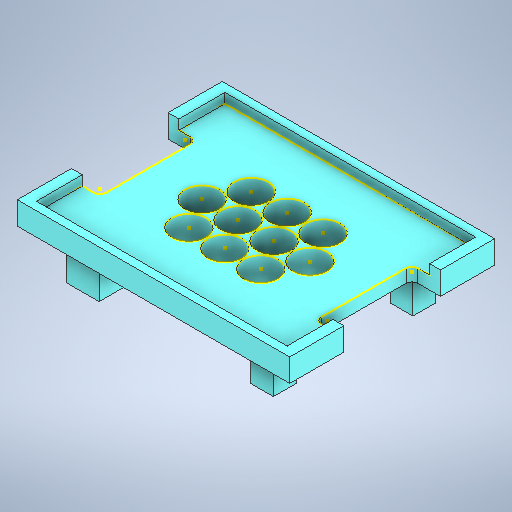
# Autodesk Inventor part: PILLARSCELLCASE18650
Saved by Autodesk Inventor 2025.2 (Build 292293000, 293)
## iProperties
Created: 2024-11-21
Part Number: PILLARSCELLCASE18650
Material: Generic
Document SubType Name: Modeling
Designer: cbast
Density: 1 g/cm^3
Appearance: Default
Mass: 190.937 g
Surface Area: 666.623 cm^2
Volume: 190.937 cm^3
Author: cbast
## iProperties of the stored document BatteryCasev1_3DPrint.ipt
Created: 2025-01-30
Part Number: BatteryCasev1_3DPrint
Material: Generic
Document SubType Name: Modeling
Designer: cbast
Density: 1 g/cm^3
Appearance: Default
Author: cbast
Autodesk Inventor part; units mm, degrees
ref_plane "YZ Plane" through (0, 0, 0) normal (1, 0, 0) x (0, 1, 0)
ref_plane "XZ Plane" through (0, 0, 0) normal (0, 1, 0) x (-1, 0, 0)
ref_plane "XY Plane" through (0, 0, 0) normal (0, 0, 1) x (1, 0, 0)
sketch "Sketch1" plane through (0, 0, 0) normal (0, 1, 0) x (-1, 0, 0)
  circle A0 centre (0, 0) radius 10.5
  circle A1 centre (22, 0) radius 10.5
  circle A2 centre (-22, 0) radius 10.5
  circle A3 centre (-11, 19.0526) radius 10.5
  circle A4 centre (11, 19.0526) radius 10.5
  circle A5 centre (33, 19.0526) radius 10.5
  circle A6 centre (11, -19.0526) radius 10.5
  circle A7 centre (33, -19.0526) radius 10.5
  circle A8 centre (-11, -19.0526) radius 10.5
  circle A9 centre (44, 0) radius 10.5
  line L0 (0, 0) -> (-32.9562, 0) construction
  line L1 (-32.9562, 0) -> (61.076, 0) construction
  circle A10 centre (0, 0) radius 11.5 construction
  circle A11 centre (-22, 0) radius 11.5 construction
  circle A12 centre (-11, -19.0526) radius 11.5 construction
  circle A13 centre (11, -19.0526) radius 11.5 construction
  circle A14 centre (33, -19.0526) radius 11.5 construction
  circle A15 centre (44, 0) radius 11.5 construction
  circle A16 centre (22, 0) radius 11.5 construction
  circle A17 centre (33, 19.0526) radius 11.5 construction
  circle A18 centre (11, 19.0526) radius 11.5 construction
  circle A19 centre (-11, 19.0526) radius 11.5 construction
  circle A20 centre (44, 0) radius 12.5 construction
  circle A21 centre (33, -19.0526) radius 12.5 construction
  circle A22 centre (11, -19.0526) radius 12.5 construction
  circle A23 centre (-11, -19.0526) radius 12.5 construction
  circle A24 centre (-22, 0) radius 12.5 construction
  circle A25 centre (-11, 19.0526) radius 12.5 construction
  circle A26 centre (11, 19.0526) radius 12.5 construction
  circle A27 centre (33, 19.0526) radius 12.5 construction
  circle A28 centre (0, 0) radius 12.5 construction
  circle A29 centre (22, 0) radius 12.5 construction
  arc A30 (43.6417, -12.4949) -> (43.6417, 12.4949) centre (43.6417, 0) ccw
  arc A31 (43.6417, 12.4949) -> (22, 24.9897) centre (33, 19.0526) ccw
  arc A32 (22, 24.9897) -> (0, 24.9897) centre (11, 19.0526) ccw
  arc A33 (0, 24.9897) -> (-21.6417, 12.4949) centre (-11, 19.0526) ccw
  arc A34 (-21.6417, 12.4949) -> (-21.6417, -12.4949) centre (-22, 0) ccw
  arc A35 (-21.6417, -12.4949) -> (0, -24.9897) centre (-11, -19.0526) ccw
  arc A36 (0, -24.9897) -> (22, -24.9897) centre (11, -19.0526) ccw
  arc A37 (22, -24.9897) -> (43.6417, -12.4949) centre (33, -19.0526) ccw
  point P0 (28.893, 7.4235)
  dimension "d0" = 21
  dimension "d2" = 21
  dimension "d4" = 21
  dimension "d6" = 21
  dimension "d8" = 21
  dimension "d10" = 21
  dimension "d11" = 21
  dimension "d13" = 21
  dimension "d14" = 21
  dimension "d53" = 21
  dimension "d91" = 1
  dimension "d144" = 23
  dimension "d145" = 23
  dimension "d146" = 23
  dimension "d147" = 23
  dimension "d148" = 23
  dimension "d149" = 23
  dimension "d150" = 23
  dimension "d151" = 23
  dimension "d152" = 23
  dimension "d153" = 23
  dimension "d154" = 25
  dimension "d155" = 25
  dimension "d156" = 25
  dimension "d157" = 25
  dimension "d158" = 25
  dimension "d159" = 25
  dimension "d160" = 25
  dimension "d161" = 25
  dimension "d162" = 25
  dimension "d163" = 25
  constraints: 38 centre point, 32 point on circle, 22 coincident, 16 tangent, 9 concentric, 4 end point, 2 point on line, 1 horizontal
  measures "d0" diameter of A0
  measures "d2" diameter of A1
  measures "d4" diameter of A2
  measures "d6" diameter of A3
  measures "d8" diameter of A4
  measures "d10" diameter of A5
  measures "d11" diameter of A6
  measures "d13" diameter of A7
  measures "d14" diameter of A8
  measures "d53" diameter of A9
  measures "d144" diameter of A10
  measures "d145" diameter of A11
  measures "d146" diameter of A12
  measures "d147" diameter of A13
  measures "d148" diameter of A14
  measures "d149" diameter of A15
  measures "d150" diameter of A16
  measures "d151" diameter of A17
  measures "d152" diameter of A18
  measures "d153" diameter of A19
  measures "d154" diameter of A20
  measures "d155" diameter of A21
  measures "d156" diameter of A22
  measures "d157" diameter of A23
  measures "d158" diameter of A24
  measures "d159" diameter of A25
  measures "d160" diameter of A26
  measures "d161" diameter of A27
  measures "d162" diameter of A28
  measures "d163" diameter of A29
extrude "Extrusion1" add sketch "Sketch1" along normal blind 15
sketch "Sketch4" plane through (0, 15, 0) normal (0, 1, 0) x (1, 0, 0)
  circle A0 centre (-33, 19.0526) radius 10.5 projected
  circle A1 centre (-44, 0) radius 10.5 projected
  circle A2 centre (-44, 0) radius 10.5 projected
  circle A3 centre (11, 19.0526) radius 10.5 projected
  circle A4 centre (-33, 19.0526) radius 10.5 projected
  circle A5 centre (-11, 19.0526) radius 10.5 projected
  circle A6 centre (-33, -19.0526) radius 10.5 projected
  circle A7 centre (-11, -19.0526) radius 10.5 projected
  circle A8 centre (11, -19.0526) radius 10.5 projected
  circle A9 centre (22, 0) radius 10.5 projected
  circle A10 centre (-22, 0) radius 10.5 projected
  circle A11 centre (0, 0) radius 10.5 projected
  line L0 (0, 0) -> (-11, 0) construction
  line L1 (-87.7, 57.7) -> (65.7, 57.7)
  line L2 (65.7, 57.7) -> (65.7, -57.7)
  line L3 (65.7, -57.7) -> (-87.7, -57.7)
  line L4 (-87.7, -57.7) -> (-87.7, 57.7)
  line L5 (-87.7, 57.7) -> (65.7, -57.7) construction
  line L6 (65.7, 57.7) -> (-87.7, -57.7) construction
  arc A12 (0, 24.9897) -> (-22, 24.9897) centre (-11, 19.0526) ccw projected
  arc A13 (21.6417, 12.4949) -> (0, 24.9897) centre (11, 19.0526) ccw projected
  arc A14 (21.6417, -12.4949) -> (21.6417, 12.4949) centre (22, 0) ccw projected
  arc A15 (0, -24.9897) -> (21.6417, -12.4949) centre (11, -19.0526) ccw projected
  arc A16 (-22, -24.9897) -> (0, -24.9897) centre (-11, -19.0526) ccw projected
  arc A17 (-43.6417, -12.4949) -> (-22, -24.9897) centre (-33, -19.0526) ccw projected
  circle A18 centre (-33, 19.0526) radius 12.5 construction
  arc A19 (-43.6417, 12.4949) -> (-43.6417, -12.4949) centre (-43.6417, 0) ccw projected
  arc A20 (-22, 24.9897) -> (-43.6417, 12.4949) centre (-33, 19.0526) ccw projected
  arc A21 (0, 24.9897) -> (-22, 24.9897) centre (-11, 19.0526) ccw
  arc A22 (21.6417, 12.4949) -> (0, 24.9897) centre (11, 19.0526) ccw
  arc A23 (21.6417, -12.4949) -> (21.6417, 12.4949) centre (22, 0) ccw
  arc A24 (0, -24.9897) -> (21.6417, -12.4949) centre (11, -19.0526) ccw
  arc A25 (-22, -24.9897) -> (0, -24.9897) centre (-11, -19.0526) ccw
  arc A26 (-43.6417, -12.4949) -> (-22, -24.9897) centre (-33, -19.0526) ccw
  arc A27 (-43.6417, 12.4949) -> (-43.6417, -12.4949) centre (-43.6417, 0) ccw
  arc A28 (-22, 24.9897) -> (-43.6417, 12.4949) centre (-33, 19.0526) ccw
  line L7 (-11.5, 0) -> (-10.5, 0) construction
  point P0 (-17.0502, -21.4927)
  point P1 (-17.0502, -11.5134)
  point P2 (-17.0502, -8.8009)
  point P3 (-17.0502, 8.8009)
  point P4 (-17.0502, 11.5134)
  point P5 (-17.0502, 21.4927)
  point P6 (-2.0059, 21.4927)
  point P7 (-2.0059, -11.5134)
  point P8 (-2.0059, -8.8009)
  point P9 (-2.0059, 8.8009)
  point P10 (-2.0059, 11.5134)
  point P11 (-2.0059, -21.4927)
  dimension "d104" = 153.4
  dimension "d164" = 115.4
  constraints: 16 end point, 16 point on circle, 8 centre point, 8 concentric, 3 midpoint, 2 horizontal, 2 parallel, 1 perpendicular, 1 point on line, 4 other
  measures "d104" distance of L2.end L3.end
  measures "d164" distance of L1.end L2.end
extrude "Extrusion7" add sketch "Sketch4" against normal blind 8 contours L1 L2 L3 L4
sketch "Sketch5" plane through (0, 15, 0) normal (0, 1, 0) x (1, 0, 0)
  line L0 (-87.7, -57.7) -> (65.7, -57.7) projected
  line L1 (65.7, -57.7) -> (65.7, 57.7) projected
  line L2 (65.7, 57.7) -> (-87.7, 57.7) projected
  line L3 (-87.7, 57.7) -> (-87.7, -57.7) projected
  circle A0 centre (-44, 0) radius 10.5 projected
  circle A1 centre (11, 19.0526) radius 10.5 projected
  circle A2 centre (-33, 19.0526) radius 10.5 projected
  circle A3 centre (-11, 19.0526) radius 10.5 projected
  circle A4 centre (-33, -19.0526) radius 10.5 projected
  circle A5 centre (-11, -19.0526) radius 10.5 projected
  circle A6 centre (11, -19.0526) radius 10.5 projected
  circle A7 centre (22, 0) radius 10.5 projected
  circle A8 centre (-22, 0) radius 10.5 projected
  circle A9 centre (0, 0) radius 10.5 projected
  line L4 (-87.7, 57.7) -> (65.7, 57.7)
  line L5 (65.7, 57.7) -> (65.7, -57.7)
  line L6 (65.7, -57.7) -> (-87.7, -57.7)
  line L7 (-87.7, -57.7) -> (-87.7, 57.7)
  line L8 (-94.3464, -62.7) -> (72.3464, -62.7)
  line L9 (72.3464, -62.7) -> (72.3464, 62.7)
  line L10 (72.3464, 62.7) -> (-94.3464, 62.7)
  line L11 (-94.3464, 62.7) -> (-94.3464, -62.7)
  line L12 (-94.3464, -62.7) -> (72.3464, 62.7) construction
  line L13 (72.3464, -62.7) -> (-94.3464, 62.7) construction
  point P0 (66.922, -57.45)
  point P1 (-11, 0)
  dimension "d169" = 5
  dimension "d170" = 6.6464
  dimension "d171" = 166.6929
  dimension "d172" = 125.4
  dimension "d221" = 6.6464
  constraints: 20 end point, 4 parallel, 4 point on line, 2 horizontal, 2 midpoint, 2 perpendicular
  measures "d169" distance between parallel lines of L10 L4
  measures "d170" distance between parallel lines of L9 L5
  measures "d171" distance of L9.end L10.end
  measures "d172" distance of L10.end L8.start
  measures "d221" distance between parallel lines of L3 L11
extrude "Extrusion8" add sketch "Sketch5" along normal blind 6 and the other way blind 8 contours L11 L10 L9 L8
sketch "Sketch6" plane through (0, 15, 0) normal (0, 1, 0) x (1, 0, 0)
  line L0 (58.472, 57.1514) -> (58.472, 25.95) construction
  line L1 (58.472, 25.95) -> (65.7, 25.95) construction
  line L2 (-80.472, -57.7) -> (-80.472, -25.95) construction
  line L3 (-80.472, -25.95) -> (-87.7, -25.95) construction
  circle A0 centre (58.472, 25.95) radius 3.615
  circle A1 centre (58.472, -25.95) radius 3.615
  circle A2 centre (-80.472, -25.95) radius 3.615
  circle A3 centre (-80.472, 25.95) radius 3.615
  line L4 (72.3464, -62.7) -> (72.3464, 62.7) projected
  line L5 (72.3464, 62.7) -> (-94.3464, 62.7) projected
  line L6 (-94.3464, 62.7) -> (-94.3464, -62.7) projected
  line L7 (-94.3464, -62.7) -> (72.3464, -62.7) projected
  line L8 (-87.7, -57.7) -> (-87.7, 57.7) projected
  line L9 (-87.7, 57.7) -> (65.7, 57.7) projected
  line L10 (65.7, 57.7) -> (65.7, -57.7) projected
  line L11 (65.7, -57.7) -> (-87.7, -57.7) projected
  line L12 (-87.7, -57.7) -> (65.7, -57.7) projected
  line L13 (65.7, -57.7) -> (65.7, 57.7) projected
  line L14 (65.7, 57.7) -> (-87.7, 57.7) projected
  line L15 (-87.7, 57.7) -> (-87.7, -57.7) projected
  circle A4 centre (-44, 0) radius 10.5 projected
  circle A5 centre (11, 19.0526) radius 10.5 projected
  circle A6 centre (-33, 19.0526) radius 10.5 projected
  circle A7 centre (-11, 19.0526) radius 10.5 projected
  circle A8 centre (-33, -19.0526) radius 10.5 projected
  circle A9 centre (-11, -19.0526) radius 10.5 projected
  circle A10 centre (11, -19.0526) radius 10.5 projected
  circle A11 centre (22, 0) radius 10.5 projected
  circle A12 centre (-22, 0) radius 10.5 projected
  circle A13 centre (0, 0) radius 10.5 projected
  line L16 (-87.7, 57.7) -> (65.7, 57.7)
  line L17 (65.7, 57.7) -> (65.7, -57.7)
  line L18 (65.7, -57.7) -> (-87.7, -57.7)
  line L19 (-87.7, -57.7) -> (-87.7, 57.7)
  dimension "d123" = 7.23
  dimension "d124" = 7.23
  dimension "d125" = 7.23
  dimension "d140" = 7.23
  dimension "d179" = 31.75
  dimension "d180" = 7.228
  dimension "d181" = 7.228
  dimension "d182" = 31.75
  dimension "d183" = 31.75
  dimension "d184" = 7.228
  dimension "d185" = 7.228
  dimension "d186" = 31.75
  constraints: 16 end point, 4 centre point, 2 coincident, 2 parallel, 1 horizontal, 1 perpendicular
  measures "d123" diameter of A0
  measures "d124" diameter of A1
  measures "d125" diameter of A2
  measures "d140" diameter of A3
  measures "d179" distance from line of A3.centre L16
  measures "d180" distance from line of A3.centre L15
  measures "d181" distance from line of A2.centre L8
  measures "d182" distance from line of L2.end L18
  measures "d183" distance from line of L12 A1.centre
  measures "d184" distance from line of L17 A1.centre
  measures "d185" distance from line of L17 L0.end
  measures "d186" distance from line of L16 L0.end
extrude "Extrusion6" cut sketch "Sketch6" against normal through all contours A0 | A1 | A2 | A3
sketch "Sketch7" plane through (-94.3464, 7, 62.7) normal (-1, 0, 0) x (0, 0, 1)
  line L0 (-120.4, 8) -> (-5, 8) projected
  line L1 (0, 0) -> (-125.4, 0) projected
  line L2 (-125.4, 14) -> (0, 14) projected
  line L3 (-92.265, 8) -> (-85.035, 8) projected
  line L4 (-40.365, 8) -> (-33.135, 8) projected
  line L5 (-92.265, 8) -> (-33.135, 8)
  line L6 (-33.135, 8) -> (-33.135, 14)
  line L7 (-33.135, 14) -> (-92.265, 14)
  line L8 (-92.265, 14) -> (-92.265, 8)
  point P0 (-62.7, -7)
  constraints: 8 end point, 2 parallel, 1 horizontal, 1 perpendicular, 1 point on line
extrude "Extrusion9" cut sketch "Sketch7" against normal through all
sketch "Sketch10" plane through (0, 7, 0) normal (0, -1, 0) x (1, 0, 0)
  circle A0 centre (-80.472, 25.95) radius 3.615 projected
  circle A1 centre (58.472, 25.95) radius 3.615 projected
  circle A2 centre (-80.472, -25.95) radius 3.615 projected
  circle A3 centre (58.472, -25.95) radius 3.615 projected
  line L0 (72.3464, -62.7) -> (72.3464, 62.7) projected
  line L1 (72.3464, 62.7) -> (-94.3464, 62.7) projected
  line L2 (-94.3464, 62.7) -> (-94.3464, -62.7) projected
  line L3 (-94.3464, -62.7) -> (72.3464, -62.7) projected
  arc A4 (-43.6417, -12.4949) -> (-22, -24.9897) centre (-33, -19.0526) ccw projected
  arc A5 (-43.6417, 12.4949) -> (-43.6417, -12.4949) centre (-43.6417, 0) ccw projected
  arc A6 (-22, 24.9897) -> (-43.6417, 12.4949) centre (-33, 19.0526) ccw projected
  arc A7 (0, 24.9897) -> (-22, 24.9897) centre (-11, 19.0526) ccw projected
  arc A8 (21.6417, 12.4949) -> (0, 24.9897) centre (11, 19.0526) ccw projected
  arc A9 (21.6417, -12.4949) -> (21.6417, 12.4949) centre (22, 0) ccw projected
  arc A10 (0, -24.9897) -> (21.6417, -12.4949) centre (11, -19.0526) ccw projected
  arc A11 (-22, -24.9897) -> (0, -24.9897) centre (-11, -19.0526) ccw projected
  line L4 (-94.3464, 62.7) -> (-64.3464, 62.7) construction
  line L5 (-94.3464, 62.7) -> (-94.3464, 42.7) construction
  line L6 (-94.3464, 42.7) -> (-64.3464, 42.7) construction
  line L7 (-74.3464, 52.7) -> (-54.3464, 52.7)
  line L8 (-54.3464, 52.7) -> (-54.3464, 32.7)
  line L9 (-54.3464, 32.7) -> (-74.3464, 32.7)
  line L10 (-74.3464, 32.7) -> (-74.3464, 52.7)
  line L11 (-74.3464, 52.7) -> (-54.3464, 32.7) construction
  line L12 (-54.3464, 52.7) -> (-74.3464, 32.7) construction
  line L13 (-71.8464, 50.2) -> (-56.8464, 50.2)
  line L14 (-56.8464, 50.2) -> (-56.8464, 35.2)
  line L15 (-56.8464, 35.2) -> (-71.8464, 35.2)
  line L16 (-71.8464, 35.2) -> (-71.8464, 50.2)
  line L17 (-71.8464, 50.2) -> (-56.8464, 35.2) construction
  line L18 (-56.8464, 50.2) -> (-71.8464, 35.2) construction
  line L19 (-94.3464, 0) -> (72.3464, 0) construction
  line L20 (-74.3464, -52.7) -> (-54.3464, -52.7)
  line L21 (-54.3464, -52.7) -> (-54.3464, -32.7)
  line L22 (-54.3464, -32.7) -> (-74.3464, -32.7)
  line L23 (-74.3464, -32.7) -> (-74.3464, -52.7)
  line L24 (-74.3464, -52.7) -> (-54.3464, -32.7) construction
  line L25 (-54.3464, -52.7) -> (-74.3464, -32.7) construction
  line L26 (-71.8464, -50.2) -> (-56.8464, -50.2)
  line L27 (-56.8464, -50.2) -> (-56.8464, -35.2)
  line L28 (-56.8464, -35.2) -> (-71.8464, -35.2)
  line L29 (-71.8464, -35.2) -> (-71.8464, -50.2)
  line L30 (-71.8464, -50.2) -> (-56.8464, -35.2) construction
  line L31 (-56.8464, -50.2) -> (-71.8464, -35.2) construction
  line L32 (72.3464, 62.7) -> (42.3464, 62.7) construction
  line L33 (42.3464, 62.7) -> (42.3464, 42.7) construction
  line L34 (35.3464, 49.7) -> (49.3464, 49.7)
  line L35 (49.3464, 49.7) -> (49.3464, 35.7)
  line L36 (49.3464, 35.7) -> (35.3464, 35.7)
  line L37 (35.3464, 35.7) -> (35.3464, 49.7)
  line L38 (35.3464, 49.7) -> (49.3464, 35.7) construction
  line L39 (49.3464, 49.7) -> (35.3464, 35.7) construction
  line L40 (35.3464, -49.7) -> (49.3464, -49.7)
  line L41 (49.3464, -49.7) -> (49.3464, -35.7)
  line L42 (49.3464, -35.7) -> (35.3464, -35.7)
  line L43 (35.3464, -35.7) -> (35.3464, -49.7)
  line L44 (35.3464, -49.7) -> (49.3464, -35.7) construction
  line L45 (49.3464, -49.7) -> (35.3464, -35.7) construction
  line L46 (42.3464, -42.7) -> (42.3464, -62.7) construction
  line L47 (42.3464, -42.7) -> (72.3464, -42.7) construction
  line L48 (-64.3464, -42.7) -> (-64.3464, -62.7) construction
  line L49 (-64.3464, -42.7) -> (-94.3464, -42.7) construction
  point P0 (0, 0)
  dimension "d209" = 30
  dimension "d210" = 20
  dimension "d211" = 20
  dimension "d212" = 20
  dimension "d213" = 15
  dimension "d214" = 15
  dimension "d215" = 30
  dimension "d216" = 20
  dimension "d217" = 14
  dimension "d218" = 14
  dimension "d224" = 30
  dimension "d225" = 30
  dimension "d226" = 20
  dimension "d227" = 20
  constraints: 92 end point, 14 symmetric about line, 8 midpoint, 8 point on line, 7 parallel, 6 perpendicular, 4 horizontal
  measures "d209" distance of L1.end L4.end
  measures "d210" distance of L1.end L5.end
  measures "d211" distance of L8.end L9.end
  measures "d212" distance of L7.end L8.end
  measures "d213" distance of L14.end L15.end
  measures "d214" distance of L13.end L14.end
  measures "d215" distance of L0.end L32.end
  measures "d216" distance of L32.end L33.end
  measures "d217" distance of L35.end L36.end
  measures "d218" distance of L34.end L35.end
  measures "d224" distance of L48.start L49.end
  measures "d225" distance of L46.start L47.end
  measures "d226" distance of L46.start L46.end
  measures "d227" distance of L48.start L48.end
extrude "Extrusion11" add sketch "Sketch10" along normal blind 25 contours L7 L8 L9 L10 | L23 L22 L21 L20 | L34 L35 L36 L37 | L43 L42 L41 L40
sketch "Sketch11" plane through (0, 7, 0) normal (0, -1, 0) x (1, 0, 0)
  line L0 (-71.8464, 50.2) -> (-71.8464, 35.2) projected
  line L1 (-71.8464, 35.2) -> (-56.8464, 35.2) projected
  line L2 (-56.8464, 35.2) -> (-56.8464, 50.2) projected
  line L3 (-56.8464, 50.2) -> (-71.8464, 50.2) projected
  line L4 (-71.8464, 50.2) -> (-56.8464, 50.2)
  line L5 (-56.8464, 50.2) -> (-56.8464, 35.2)
  line L6 (-56.8464, 35.2) -> (-71.8464, 35.2)
  line L7 (-71.8464, 35.2) -> (-71.8464, 50.2)
  line L8 (-56.8464, -35.2) -> (-71.8464, -35.2) projected
  line L9 (-71.8464, -35.2) -> (-71.8464, -50.2) projected
  line L10 (-71.8464, -50.2) -> (-56.8464, -50.2) projected
  line L11 (-56.8464, -50.2) -> (-56.8464, -35.2) projected
  line L12 (-71.8464, -35.2) -> (-56.8464, -35.2)
  line L13 (-56.8464, -35.2) -> (-56.8464, -50.2)
  line L14 (-56.8464, -50.2) -> (-71.8464, -50.2)
  line L15 (-71.8464, -50.2) -> (-71.8464, -35.2)
  point P0 (0, 0)
  constraints: 16 end point, 4 parallel, 2 horizontal, 2 perpendicular
extrude "Extrusion12" add sketch "Sketch11" along normal up to surface (12.5 mm away)
sketch "Sketch13" plane through (0, 7, 0) normal (0, -1, 0) x (1, 0, 0)
  line L0 (35.3464, 35.7) -> (35.3464, 49.7) projected
  line L1 (35.3464, 49.7) -> (49.3464, 49.7) projected
  line L2 (49.3464, 49.7) -> (49.3464, 35.7) projected
  line L3 (49.3464, 35.7) -> (35.3464, 35.7) projected
  line L4 (-74.3464, -32.7) -> (-54.3464, -32.7) projected
  line L5 (-54.3464, -32.7) -> (-54.3464, -52.7) projected
  line L6 (-54.3464, -52.7) -> (-74.3464, -52.7) projected
  line L7 (-74.3464, -52.7) -> (-74.3464, -32.7) projected
  line L8 (35.3464, -49.7) -> (35.3464, -35.7) projected
  line L9 (35.3464, -35.7) -> (49.3464, -35.7) projected
  line L10 (49.3464, -35.7) -> (49.3464, -49.7) projected
  line L11 (49.3464, -49.7) -> (35.3464, -49.7) projected
  line L12 (-74.3464, 32.7) -> (-74.3464, 52.7) projected
  line L13 (-74.3464, 52.7) -> (-54.3464, 52.7) projected
  line L14 (-54.3464, 52.7) -> (-54.3464, 32.7) projected
  line L15 (-54.3464, 32.7) -> (-74.3464, 32.7) projected
  circle A0 centre (-80.472, 25.95) radius 3.615 projected
  circle A1 centre (58.472, 25.95) radius 3.615 projected
  circle A2 centre (-80.472, -25.95) radius 3.615 projected
  circle A3 centre (58.472, -25.95) radius 3.615 projected
  line L16 (72.3464, -62.7) -> (72.3464, 62.7) projected
  line L17 (72.3464, 62.7) -> (-94.3464, 62.7) projected
  line L18 (-94.3464, 62.7) -> (-94.3464, -62.7) projected
  line L19 (-94.3464, -62.7) -> (72.3464, -62.7) projected
  arc A4 (-43.6417, -12.4949) -> (-22, -24.9897) centre (-33, -19.0526) ccw projected
  arc A5 (-43.6417, 12.4949) -> (-43.6417, -12.4949) centre (-43.6417, 0) ccw projected
  arc A6 (-22, 24.9897) -> (-43.6417, 12.4949) centre (-33, 19.0526) ccw projected
  arc A7 (0, 24.9897) -> (-22, 24.9897) centre (-11, 19.0526) ccw projected
  arc A8 (21.6417, 12.4949) -> (0, 24.9897) centre (11, 19.0526) ccw projected
  arc A9 (21.6417, -12.4949) -> (21.6417, 12.4949) centre (22, 0) ccw projected
  arc A10 (0, -24.9897) -> (21.6417, -12.4949) centre (11, -19.0526) ccw projected
  arc A11 (-22, -24.9897) -> (0, -24.9897) centre (-11, -19.0526) ccw projected
  line L20 (-94.3464, 29.565) -> (-80.472, 29.565)
  line L21 (-76.857, 25.95) -> (-76.857, -25.95)
  line L22 (-80.472, -29.565) -> (-94.3464, -29.565)
  line L23 (-94.3464, -29.565) -> (-94.3464, 29.565)
  line L24 (-11, 27.2798) -> (-11, -25.95) construction
  line L25 (72.3464, 29.565) -> (58.472, 29.565)
  line L26 (54.857, 25.95) -> (54.857, -25.95)
  line L27 (58.472, -29.565) -> (72.3464, -29.565)
  point P0 (0, 0)
  point P1 (-76.857, -29.565)
  point P2 (-76.857, 29.565)
  point P3 (54.857, -29.565)
  point P4 (54.857, 29.565)
  point P5 (58.472, -29.565)
  point P6 (72.3464, -29.565)
  point P7 (72.3464, 29.565)
  point P8 (58.472, 29.565)
  point P9 (54.857, 25.95)
  point P10 (54.857, -25.95)
  point P11 (-80.472, -29.565)
  point P12 (-76.857, -25.95)
  point P13 (-76.857, 25.95)
  point P14 (-80.472, 29.565)
  point P15 (56.3464, -28.8741)
  point P16 (56.3464, 23.0259)
  dimension "d234" = 0
  dimension "d235" = 0
  constraints: 16 end point, 8 point on circle, 4 symmetric about line, 2 parallel, 1 horizontal, 1 perpendicular, 1 point on line, 1 vertical
  measures "d234" distance edge to line of A3 L26
  measures "d235" distance edge to line of A2 L21
extrude "Extrusion14" cut sketch "Sketch13" against normal blind 10 contours L21 A2 L22 L18 L20 A0 | L16 L27 A3 L26 A1 L25
sketch "Sketch14" plane through (0, 15, 0) normal (0, 1, 0) x (1, 0, 0)
  line L0 (65.7, -29.565) -> (58.472, -29.565) projected
  arc A0 (54.857, -25.95) -> (58.472, -29.565) centre (58.472, -25.95) ccw projected
  line L1 (54.857, -25.95) -> (54.857, 25.95) projected
  arc A1 (58.472, 29.565) -> (54.857, 25.95) centre (58.472, 25.95) ccw projected
  line L2 (58.472, 29.565) -> (65.7, 29.565) projected
  line L3 (65.7, 29.565) -> (65.7, 57.7) projected
  line L4 (65.7, 57.7) -> (-87.7, 57.7) projected
  line L5 (-87.7, 57.7) -> (-87.7, 29.565) projected
  line L6 (-87.7, 29.565) -> (-80.472, 29.565) projected
  arc A2 (-76.857, 25.95) -> (-80.472, 29.565) centre (-80.472, 25.95) ccw projected
  line L7 (-76.857, 25.95) -> (-76.857, -25.95) projected
  arc A3 (-80.472, -29.565) -> (-76.857, -25.95) centre (-80.472, -25.95) ccw projected
  line L8 (-80.472, -29.565) -> (-87.7, -29.565) projected
  line L9 (-87.7, -29.565) -> (-87.7, -57.7) projected
  line L10 (-87.7, -57.7) -> (65.7, -57.7) projected
  line L11 (65.7, -57.7) -> (65.7, -29.565) projected
  circle A4 centre (-44, 0) radius 10.5 projected
  circle A5 centre (11, 19.0526) radius 10.5 projected
  circle A6 centre (-33, 19.0526) radius 10.5 projected
  circle A7 centre (-11, 19.0526) radius 10.5 projected
  circle A8 centre (-33, -19.0526) radius 10.5 projected
  circle A9 centre (-11, -19.0526) radius 10.5 projected
  circle A10 centre (11, -19.0526) radius 10.5 projected
  circle A11 centre (22, 0) radius 10.5 projected
  circle A12 centre (-22, 0) radius 10.5 projected
  circle A13 centre (0, 0) radius 10.5 projected
  line L12 (-11.5, 0) -> (-10.5, 0) construction
  constraints: 2 end point, 2 horizontal alignment, 1 horizontal, 2 other
body "Solid1"
